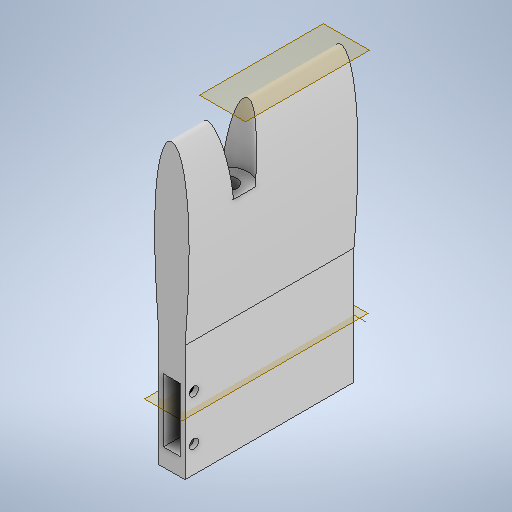
# Autodesk Inventor part: OuterTailLeft
Saved by Autodesk Inventor 2025.2 (Build 292293000, 293)
## iProperties
Created: 2025-03-03
Part Number: OuterTailLeft
Material: Generic
Document SubType Name: Modeling
Designer: georg
Density: 1 g/cm^3
Appearance: Default
Author: georg
Autodesk Inventor part; units mm, degrees
ref_plane "YZ Plane" through (0, 0, 0) normal (1, 0, 0) x (0, 1, 0)
ref_plane "Work Plane1" through (0, 0, 241.1984) normal (0, 0, 1) x (1, 0, 0)
sketch "Sketch1" plane through (0, 0, 241.1984) normal (0, 0, 1) x (1, 0, 0)
  line L0 (-7.0407, -203.2) -> (7.0407, -203.2)
  line L1 (-9.3456, -120.638) -> (-9.3456, -203.2)
  line L2 (-9.3456, -203.2) -> (9.3456, -203.2)
  line L3 (9.3456, -203.2) -> (9.3456, -120.638)
  spline S0 degree 5 poles (9.3456, -120.638) (9.3457, -120.6362) (9.3974, -120.0068) (9.5, -118.7472) (9.6516, -116.8541) (9.8495, -114.3238) (10.0866, -111.1538) (10.3164, -107.9748) (10.5349, -104.7893) (10.7445, -101.6008) (10.942, -98.4123) (11.1277, -95.2267) (11.3009, -92.0477) (11.4615, -88.8777) (11.6069, -85.7208) (11.739, -82.5791) (11.8548, -79.4563) (11.9554, -76.3556) (12.039, -73.2792) (12.1057, -70.2316) (12.1549, -67.2141) (12.1854, -64.2311) (12.198, -61.2847) (12.1911, -58.378) (12.1652, -55.5142) (12.1197, -52.6956) (12.0539, -49.9253) (11.9681, -47.2063) (11.8622, -44.5404) (11.7355, -41.9312) (11.589, -39.3806) (11.4216, -36.8917) (11.2342, -34.4665) (11.0264, -32.1073) (10.7996, -29.817) (10.5524, -27.5973) (10.2861, -25.4503) (10.0015, -23.3788) (9.698, -21.3841) (9.3765, -19.469) (9.0379, -17.6343) (8.682, -15.8826) (8.3103, -14.2152) (7.9227, -12.634) (7.5202, -11.1404) (7.103, -9.7353) (6.6725, -8.4212) (6.2284, -7.198) (5.7722, -6.0677) (5.3036, -5.0307) (4.8237, -4.0882) (4.3332, -3.2402) (3.831, -2.4886) (3.3186, -1.832) (2.7948, -1.2726) (2.2592, -0.8103) (1.7116, -0.4465) (1.151, -0.1846) (0.5803, -0.0264) (0, 0.026) (-0.5803, -0.0264) (-1.151, -0.1846) (-1.7116, -0.4465) (-2.2592, -0.8103) (-2.7948, -1.2726) (-3.3186, -1.832) (-3.831, -2.4886) (-4.3332, -3.2402) (-4.8237, -4.0882) (-5.3036, -5.0307) (-5.7722, -6.0677) (-6.2284, -7.198) (-6.6725, -8.4212) (-7.103, -9.7353) (-7.5202, -11.1404) (-7.9227, -12.634) (-8.3103, -14.2152) (-8.682, -15.8826) (-9.0379, -17.6343) (-9.3765, -19.469) (-9.698, -21.3841) (-10.0015, -23.3788) (-10.2861, -25.4503) (-10.5524, -27.5973) (-10.7996, -29.817) (-11.0264, -32.1073) (-11.2342, -34.4665) (-11.4216, -36.8917) (-11.589, -39.3806) (-11.7355, -41.9312) (-11.8622, -44.5404) (-11.9681, -47.2063) (-12.0539, -49.9253) (-12.1197, -52.6956) (-12.1652, -55.5142) (-12.1911, -58.378) (-12.198, -61.2847) (-12.1854, -64.2311) (-12.1549, -67.2141) (-12.1057, -70.2316) (-12.039, -73.2792) (-11.9554, -76.3556) (-11.8548, -79.4563) (-11.739, -82.5791) (-11.6069, -85.7208) (-11.4615, -88.8777) (-11.3009, -92.0477) (-11.1277, -95.2267) (-10.942, -98.4123) (-10.7445, -101.6008) (-10.5349, -104.7893) (-10.3164, -107.9748) (-10.0866, -111.1538) (-9.8495, -114.3238) (-9.6516, -116.8541) (-9.5, -118.7472) (-9.3974, -120.0068) (-9.3457, -120.6362) (-9.3456, -120.638) knots 0.207665 0.207665 0.207665 0.207665 0.207665 0.207665 0.207683 0.214076 0.220484 0.226904 0.233333 0.239767 0.246204 0.25264 0.259072 0.265497 0.271912 0.278314 0.284699 0.291064 0.297407 0.303723 0.310011 0.316266 0.322485 0.328666 0.334804 0.340898 0.346943 0.352937 0.358876 0.364757 0.370576 0.376331 0.382017 0.387632 0.393172 0.398634 0.404014 0.409309 0.414515 0.419627 0.424644 0.42956 0.434371 0.439075 0.443667 0.448142 0.452498 0.456729 0.460831 0.464802 0.468638 0.472335 0.475892 0.479309 0.482586 0.485731 0.488751 0.491664 0.494492 0.497262 0.5 0.502738 0.505508 0.508336 0.511249 0.514269 0.517414 0.520691 0.524108 0.527665 0.531362 0.535198 0.539169 0.543271 0.547502 0.551858 0.556333 0.560925 0.565629 0.57044 0.575356 0.580373 0.585485 0.590691 0.595986 0.601366 0.606828 0.612368 0.617983 0.623669 0.629424 0.635243 0.641124 0.647063 0.653057 0.659102 0.665196 0.671334 0.677515 0.683734 0.689989 0.696277 0.702593 0.708936 0.715301 0.721686 0.728088 0.734503 0.740928 0.74736 0.753796 0.760233 0.766667 0.773096 0.779516 0.785924 0.792317 0.792335 0.792335 0.792335 0.792335 0.792335 0.792335
  point P0 (0, 0)
  point P1 (9.3456, -120.638)
  point P2 (10.084, -111.1614)
  point P3 (10.3132, -107.9795)
  point P4 (10.5325, -104.7913)
  point P5 (10.7416, -101.6)
  point P6 (10.9393, -98.4087)
  point P7 (11.125, -95.2205)
  point P8 (11.2983, -92.0386)
  point P9 (11.4584, -88.8661)
  point P10 (11.6043, -85.7063)
  point P11 (11.7358, -82.562)
  point P12 (11.8518, -79.4366)
  point P13 (11.952, -76.3331)
  point P14 (12.0355, -73.2544)
  point P15 (12.102, -70.204)
  point P16 (12.1508, -67.1842)
  point P17 (12.1812, -64.1986)
  point P18 (12.1932, -61.2498)
  point P19 (12.1861, -58.3408)
  point P20 (12.1597, -55.4746)
  point P21 (12.1136, -52.6538)
  point P22 (12.0473, -49.8813)
  point P23 (11.961, -47.1601)
  point P24 (11.8543, -44.4923)
  point P25 (11.7271, -41.8809)
  point P26 (11.5796, -39.3285)
  point P27 (11.4115, -36.8377)
  point P28 (11.2231, -34.4107)
  point P29 (11.0147, -32.0499)
  point P30 (10.7865, -29.758)
  point P31 (10.5384, -27.5369)
  point P32 (10.2709, -25.3886)
  point P33 (9.9848, -23.3158)
  point P34 (9.68, -21.3202)
  point P35 (9.3572, -19.404)
  point P36 (9.0168, -17.5687)
  point P37 (8.6594, -15.8163)
  point P38 (8.2857, -14.1486)
  point P39 (7.8961, -12.5673)
  point P40 (7.4914, -11.0738)
  point P41 (7.072, -9.6695)
  point P42 (6.6387, -8.3562)
  point P43 (6.1921, -7.1348)
  point P44 (5.7329, -6.0066)
  point P45 (5.2615, -4.9727)
  point P46 (4.7787, -4.0341)
  point P47 (4.2851, -3.1919)
  point P48 (3.7809, -2.4469)
  point P49 (3.267, -1.7995)
  point P50 (2.7438, -1.2509)
  point P51 (2.2116, -0.8012)
  point P52 (1.6709, -0.4509)
  point P53 (1.1219, -0.2006)
  point P54 (0.5647, -0.0502)
  point P55 (0, 0)
  point P56 (-0.5647, -0.0502)
  point P57 (-1.1219, -0.2006)
  point P58 (-1.6709, -0.4509)
  point P59 (-2.2116, -0.8012)
  point P60 (-2.7438, -1.2509)
  point P61 (-3.267, -1.7995)
  point P62 (-3.7809, -2.4469)
  point P63 (-4.2851, -3.1919)
  point P64 (-4.7787, -4.0341)
  point P65 (-5.2615, -4.9727)
  point P66 (-5.7329, -6.0066)
  point P67 (-6.1921, -7.1348)
  point P68 (-6.6387, -8.3562)
  point P69 (-7.072, -9.6695)
  point P70 (-7.4914, -11.0738)
  point P71 (-7.8961, -12.5673)
  point P72 (-8.2857, -14.1486)
  point P73 (-8.6594, -15.8163)
  point P74 (-9.0168, -17.5687)
  point P75 (-9.3572, -19.404)
  point P76 (-9.68, -21.3202)
  point P77 (-9.9848, -23.3158)
  point P78 (-10.2709, -25.3886)
  point P79 (-10.5384, -27.5369)
  point P80 (-10.7865, -29.758)
  point P81 (-11.0147, -32.0499)
  point P82 (-11.2231, -34.4107)
  point P83 (-11.4115, -36.8377)
  point P84 (-11.5796, -39.3285)
  point P85 (-11.7271, -41.8809)
  point P86 (-11.8543, -44.4923)
  point P87 (-11.961, -47.1601)
  point P88 (-12.0473, -49.8813)
  point P89 (-12.1136, -52.6538)
  point P90 (-12.1597, -55.4746)
  point P91 (-12.1861, -58.3408)
  point P92 (-12.1932, -61.2498)
  point P93 (-12.1812, -64.1986)
  point P94 (-12.1508, -67.1842)
  point P95 (-12.102, -70.204)
  point P96 (-12.0355, -73.2544)
  point P97 (-11.952, -76.3331)
  point P98 (-11.8518, -79.4366)
  point P99 (-11.7358, -82.562)
  point P100 (-11.6043, -85.7063)
  point P101 (-11.4584, -88.8661)
  point P102 (-11.2983, -92.0386)
  point P103 (-11.125, -95.2205)
  point P104 (-10.9393, -98.4087)
  point P105 (-10.7416, -101.6)
  point P106 (-10.5325, -104.7913)
  point P107 (-10.3132, -107.9795)
  point P108 (-10.084, -111.1614)
  point P109 (-9.8461, -114.3339)
  point P110 (-9.5996, -117.4937)
  point P111 (0, -203.2)
  dimension "d2" = 203.2
  constraints: 8 end point, 2 perpendicular, 1 coincident, 1 parallel, 1 point on line, 113 other
  measures "d2" distance of point (0, -203.2) point (0, 0)
extrude "Extrusion1" add sketch "Sketch1" along normal blind 120
ref_plane "Work Plane3" through (9.5807, -152.3935, 308.473) normal (0, 0, 1) x (0, 1, 0)
ref_plane "Work Plane4" through (-0.0008, 2.54, 241.1984) normal (0, 1, 0) x (0, 0, 1)
sketch "Sketch3" plane through (-0.0008, 2.54, 241.1984) normal (0, 1, 0) x (0, 0, 1)
  circle A0 centre (80.2, 0.0008) radius 14.2875
  line L0 (120, 7.0415) -> (120, -7.0399) projected
  line L1 (-250, 20.9554) -> (-250, -20.9701)
  point P0 (-241.1984, 0.0008)
  point P1 (120, 0.0008)
  dimension "d8" = 28.575
  dimension "d15" = 330.2
  constraints: 2 end point, 1 centre point, 1 midpoint, 1 vertical, 2 other
  measures "d8" diameter of A0
  measures "d15" distance from line of L1 A0.centre
extrude "Extrusion2" cut sketch "Sketch3" against normal blind 48.004
ref_plane "Work Plane5" through (9.5807, -152.3935, 321.173) normal (0, 0, 1) x (0, 1, 0)
sketch "Sketch9" plane through (0, 0, 361.1984) normal (0, 0, 1) x (1, 0, 0)
  line L0 (6, -190.6499) -> (-6, -190.6499)
  line L1 (-6, -190.6499) -> (-6, -145.6499)
  line L2 (-6, -145.6499) -> (6, -145.6499)
  line L3 (6, -145.6499) -> (6, -190.6499)
  line L4 (6, -190.6499) -> (-6, -145.6499) construction
  line L5 (-6, -190.6499) -> (6, -145.6499) construction
  line L6 (-9.3456, -203.2) -> (9.3456, -203.2) projected
  point P0 (0, 0)
  point P1 (0, -168.1499)
  point P2 (7.0407, -203.2)
  point P3 (-6, -168.1499)
  dimension "d33" = 12
  dimension "d42" = 45
  dimension "d44" = 57.55
  constraints: 12 end point, 3 midpoint, 2 parallel, 1 horizontal, 1 perpendicular
  measures "d33" distance between parallel lines of L3 L1
  measures "d42" distance of L2.end L0.start
  measures "d44" distance between parallel lines of L6 L2
extrude "Extrusion7" cut sketch "Sketch9" against normal blind 108.5088
sketch "Sketch10" plane through (-0.0008, -45.464, 241.1984) normal (0, 1, 0) x (1, 0, 0)
  line L0 (0, 313.4381) -> (0, -192.2397) projected
  arc A0 (11.8966, -72.2865) -> (-11.895, -72.2865) centre (0.0008, -80.2) ccw projected
  arc A1 (-11.895, -88.1135) -> (11.8966, -88.1135) centre (0.0008, -80.2) ccw projected
  circle A2 centre (0.0008, -80.2) radius 6.35
  point P0 (0.0008, 241.1984)
  dimension "d39" = 12.7
  constraints: 2 vertical alignment, 1 centre point, 1 coincident
  measures "d39" diameter of A2
extrude "Extrusion8" cut sketch "Sketch10" against normal blind 121.5771
sketch "Sketch11" plane through (0, 0, 252.6896) normal (0, 0, 1) x (1, 0, 0)
  line L0 (-6, -190.6499) -> (-6, -145.6499) projected
  line L1 (-6, -145.6499) -> (6, -145.6499) projected
  line L2 (-6, -190.6499) -> (-6, -145.6499) projected
  line L3 (6, -190.6499) -> (-6, -190.6499) projected
  line L4 (6, -145.6499) -> (6, -190.6499) projected
  line L5 (6, -173.355) -> (-6, -173.355)
  line L6 (-6, -173.355) -> (-6, -150.3426)
  line L7 (-6, -150.3426) -> (6, -150.3426)
  line L8 (6, -150.3426) -> (6, -173.355)
  line L9 (-9.3456, -203.2) -> (9.3456, -203.2) projected
  point P0 (0, 0)
  dimension "d45" = 12
  dimension "d46" = 23.0124
  dimension "d47" = 52.8574
  constraints: 8 end point, 2 parallel, 2 perpendicular, 2 point on line
  measures "d45" distance of L5.start L5.end
  measures "d46" distance between parallel lines of L7 L5
  measures "d47" distance between parallel lines of L7 L9
extrude "Extrusion9" cut sketch "Sketch11" against normal blind 27.5336 contours L0 L7 L4 L5
sketch "Sketch12" plane through (0, 0, 241.1984) normal (0, 0, -1) x (-1, 0, 0)
  line L0 (-6, -150.3426) -> (6, -150.3426) projected
  line L1 (6, -150.3426) -> (6, -173.355) projected
  line L2 (-6, -173.355) -> (-6, -150.3426) projected
  line L3 (6, -173.355) -> (-6, -173.355) projected
  line L4 (6, -190.6499) -> (6, -145.6499) projected
  line L5 (-6, -146.3548) -> (6, -146.3548)
  line L6 (6, -146.3548) -> (6, -177.3428)
  line L7 (6, -177.3428) -> (-6, -177.3428)
  line L8 (-6, -177.3428) -> (-6, -146.3548)
  line L9 (-6, -146.3548) -> (6, -177.3428) construction
  line L10 (6, -146.3548) -> (-6, -177.3428) construction
  point P0 (0, 0)
  point P1 (0, -161.8488)
  dimension "d50" = 30.988
  constraints: 12 end point, 2 midpoint, 2 parallel, 1 horizontal, 1 perpendicular, 1 point on line
  measures "d50" distance of L7.end L5.start
extrude "Extrusion10" cut sketch "Sketch12" against normal blind 6.5
sketch "Sketch13" plane through (0, 0, 247.6984) normal (0, 0, -1) x (-1, 0, 0)
  circle A0 centre (4, -175.3428) radius 1.25
  circle A1 centre (-4, -175.3428) radius 1.25
  line L0 (6, -146.3548) -> (6, -177.3428) projected
  line L1 (-6, -177.3428) -> (-6, -146.3548) projected
  line L2 (6, -177.3428) -> (-6, -177.3428) projected
  point P0 (0, 0)
  dimension "d53" = 2.5
  dimension "d54" = 2.5
  dimension "d55" = 2
  dimension "d56" = 2
  dimension "d57" = 2
  dimension "d58" = 2
  constraints: 2 centre point
  measures "d53" diameter of A0
  measures "d54" diameter of A1
  measures "d55" distance from line of L0 A0.centre
  measures "d56" distance from line of L1 A1.centre
  measures "d57" distance from line of L2 A0.centre
  measures "d58" distance from line of L2 A1.centre
extrude "Extrusion11" cut sketch "Sketch13" against normal blind 22
ref_plane "Work Plane6" through (-6, -161.8488, 241.1984) normal (0, 1, 0) x (1, 0, 0)
mirror "Mirror1" about plane through (-6, -161.8488, 241.1984) normal (0, 1, 0) of "Extrusion11"
sketch "Sketch14" plane through (0, 0, 241.1984) normal (0, 0, -1) x (-1, 0, 0)
  circle A0 centre (0.0018, -25.4) radius 3.175
  circle A1 centre (0.0018, -120.269) radius 3.175
  circle A2 centre (0.0018, -72.8345) radius 3.175
  point P0 (0, 0)
  point P1 (0, 0)
  dimension "d62" = 6.35
  dimension "d63" = 6.35
  dimension "d64" = 6.35
  dimension "d66" = 25.4
  dimension "d68" = 47.4345
  dimension "d69" = 120.269
  constraints: 3 centre point, 1 coincident
  measures "d62" diameter of A0
  measures "d63" diameter of A1
  measures "d64" diameter of A2
  measures "d66" distance of point (0, 0) A0.centre
  measures "d68" distance of A1.centre A2.centre
  measures "d69" distance of A1.centre point (0, 0)
extrude "Extrusion12" cut sketch "Sketch14" against normal blind 25.4
sketch "Sketch16" plane through (9.3456, -203.2, 241.1984) normal (1, 0, 0) x (0, 0, -1)
  circle A0 centre (-113.65, 18.8976) radius 3.175
  line L0 (0, 0) -> (-120, 0) projected
  line L1 (-120, 0) -> (-120, 82.562) projected
  point P0 (241.1984, 203.2)
  dimension "d72" = 6.35
  dimension "d73" = 18.8976
  dimension "d74" = 6.35
  constraints: 1 centre point
  measures "d72" diameter of A0
  measures "d73" distance from line of A0.centre L0
  measures "d74" distance from line of L1 A0.centre
extrude "Extrusion13" cut sketch "Sketch16" against normal blind 6.35
sketch "Sketch17" plane through (9.3456, -203.2, 241.1984) normal (1, 0, 0) x (0, 0, -1)
  circle A0 centre (-113.65, 51.2064) radius 3.175
  circle A1 centre (-113.65, 18.8976) radius 3.175 projected
  line L0 (-120, 0) -> (-120, 82.562) projected
  point P0 (241.1984, 203.2)
  dimension "d77" = 6.35
  dimension "d78" = 32.3088
  dimension "d79" = 6.35
  constraints: 1 centre point
  measures "d77" diameter of A0
  measures "d78" distance of A1.centre A0.centre
  measures "d79" distance from line of L0 A0.centre
extrude "Extrusion14" cut sketch "Sketch17" against normal blind 6.35 contours A0
body "Solid1"
